Autodesk Inventor part; units mm, degrees
(part 3 of 4)
sketch "Швелер 24" plane through (0, 0, 0) normal (0, 0, 1) x (1, 0, 0)
  line L0 (-3.4674, 143.7463) -> (-3.4674, -55.2537)
  line L1 (80.9326, -75.7537) -> (-9.0674, -75.7537)
  line L2 (-9.0674, -75.7537) -> (-9.0674, 164.2463)
  line L3 (-9.0674, 164.2463) -> (80.9326, 164.2463)
  line L4 (76.9326, 154.2463) -> (7.0326, 154.2463)
  arc A0 (7.0326, 154.2463) -> (-3.4674, 143.7463) centre (7.0326, 143.7463) ccw
  arc A1 (-3.4674, -55.2537) -> (7.0326, -65.7537) centre (7.0326, -55.2537) ccw
  line L5 (7.0326, -65.7537) -> (76.9326, -65.7537)
  line L6 (80.9326, -75.7537) -> (80.9326, -69.7537)
  arc A2 (80.9326, -69.7537) -> (76.9326, -65.7537) centre (76.9326, -69.7537) ccw
  line L7 (80.9326, 164.2463) -> (80.9326, 158.2463)
  arc A3 (76.9326, 154.2463) -> (80.9326, 158.2463) centre (76.9326, 158.2463) ccw
  point P0 (39.2152, 43.3464)
  dimension "d495" = 90
  dimension "d496" = 240
  dimension "d497" = 5.6
  dimension "d498" = 10.5
  dimension "d499" = 4
  dimension "d500" = 10
  measures "d495" distance of L1.start L1.end
  measures "d496" distance of L1.end L2.end
  measures "d497" distance between parallel lines of L2 L0
  measures "d498" radius of A1
  measures "d499" radius of A2
  measures "d500" distance between parallel lines of L1 L5
sketch "Швелер 24а" plane through (0, 0, 0) normal (0, 0, 1) x (1, 0, 0)
  line L0 (-6.1145, 143.0463) -> (-6.1145, -54.5537)
  line L1 (83.2855, -75.7537) -> (-11.7145, -75.7537)
  line L2 (-11.7145, -75.7537) -> (-11.7145, 164.2463)
  line L3 (-11.7145, 164.2463) -> (83.2855, 164.2463)
  line L4 (79.2855, 153.5463) -> (4.3855, 153.5463)
  arc A0 (4.3855, 153.5463) -> (-6.1145, 143.0463) centre (4.3855, 143.0463) ccw
  arc A1 (-6.1145, -54.5537) -> (4.3855, -65.0537) centre (4.3855, -54.5537) ccw
  line L5 (4.3855, -65.0537) -> (79.2855, -65.0537)
  line L6 (83.2855, -75.7537) -> (83.2855, -69.0537)
  arc A2 (83.2855, -69.0537) -> (79.2855, -65.0537) centre (79.2855, -69.0537) ccw
  line L7 (83.2855, 164.2463) -> (83.2855, 157.5463)
  arc A3 (79.2855, 153.5463) -> (83.2855, 157.5463) centre (79.2855, 157.5463) ccw
  point P0 (39.2152, 43.3464)
  dimension "d501" = 95
  dimension "d502" = 240
  dimension "d503" = 5.6
  dimension "d504" = 10.5
  dimension "d505" = 4
  dimension "d506" = 10.7
  measures "d501" distance of L1.start L1.end
  measures "d502" distance of L1.end L2.end
  measures "d503" distance between parallel lines of L2 L0
  measures "d504" radius of A1
  measures "d505" radius of A2
  measures "d506" distance between parallel lines of L1 L5
sketch "Швелер 27" plane through (0, 0, 0) normal (0, 0, 1) x (1, 0, 0)
  line L0 (-5.8322, 157.7463) -> (-5.8322, -69.2537)
  line L1 (83.1678, -90.7537) -> (-11.8322, -90.7537)
  line L2 (-11.8322, -90.7537) -> (-11.8322, 179.2463)
  line L3 (-11.8322, 179.2463) -> (83.1678, 179.2463)
  line L4 (78.6678, 168.7463) -> (5.1678, 168.7463)
  arc A0 (5.1678, 168.7463) -> (-5.8322, 157.7463) centre (5.1678, 157.7463) ccw
  arc A1 (-5.8322, -69.2537) -> (5.1678, -80.2537) centre (5.1678, -69.2537) ccw
  line L5 (5.1678, -80.2537) -> (78.6678, -80.2537)
  line L6 (83.1678, -90.7537) -> (83.1678, -84.7537)
  arc A2 (83.1678, -84.7537) -> (78.6678, -80.2537) centre (78.6678, -84.7537) ccw
  line L7 (83.1678, 179.2463) -> (83.1678, 173.2463)
  arc A3 (78.6678, 168.7463) -> (83.1678, 173.2463) centre (78.6678, 173.2463) ccw
  point P0 (39.2152, 43.3464)
  dimension "d507" = 95
  dimension "d508" = 270
  dimension "d509" = 6
  dimension "d510" = 11
  dimension "d511" = 4.5
  dimension "d512" = 10.5
  measures "d507" distance of L1.start L1.end
  measures "d508" distance of L1.end L2.end
  measures "d509" distance between parallel lines of L2 L0
  measures "d510" radius of A1
  measures "d511" radius of A2
  measures "d512" distance between parallel lines of L1 L5
sketch "Швелер 30" plane through (0, 0, 0) normal (0, 0, 1) x (1, 0, 0)
  line L0 (-8.2439, 171.2463) -> (-8.2439, -82.7537)
  line L1 (85.2561, -105.7537) -> (-14.7439, -105.7537)
  line L2 (-14.7439, -105.7537) -> (-14.7439, 194.2463)
  line L3 (-14.7439, 194.2463) -> (85.2561, 194.2463)
  line L4 (80.2561, 183.2463) -> (3.7561, 183.2463)
  arc A0 (3.7561, 183.2463) -> (-8.2439, 171.2463) centre (3.7561, 171.2463) ccw
  arc A1 (-8.2439, -82.7537) -> (3.7561, -94.7537) centre (3.7561, -82.7537) ccw
  line L5 (3.7561, -94.7537) -> (80.2561, -94.7537)
  line L6 (85.2561, -105.7537) -> (85.2561, -99.7537)
  arc A2 (85.2561, -99.7537) -> (80.2561, -94.7537) centre (80.2561, -99.7537) ccw
  line L7 (85.2561, 194.2463) -> (85.2561, 188.2463)
  arc A3 (80.2561, 183.2463) -> (85.2561, 188.2463) centre (80.2561, 188.2463) ccw
  point P0 (39.2152, 43.3464)
  dimension "d513" = 100
  dimension "d514" = 300
  dimension "d515" = 6.5
  dimension "d516" = 12
  dimension "d517" = 5
  dimension "d518" = 11
  measures "d513" distance of L1.start L1.end
  measures "d514" distance of L1.end L2.end
  measures "d515" distance between parallel lines of L2 L0
  measures "d516" radius of A1
  measures "d517" radius of A2
  measures "d518" distance between parallel lines of L1 L5
sketch "Швелер 33" plane through (0, 0, 0) normal (0, 0, 1) x (1, 0, 0)
  line L0 (-10.7733, 184.5463) -> (-10.7733, -96.0537)
  line L1 (87.2267, -120.7537) -> (-17.7733, -120.7537)
  line L2 (-17.7733, -120.7537) -> (-17.7733, 209.2463)
  line L3 (-17.7733, 209.2463) -> (87.2267, 209.2463)
  line L4 (82.2267, 197.5463) -> (2.2267, 197.5463)
  arc A0 (2.2267, 197.5463) -> (-10.7733, 184.5463) centre (2.2267, 184.5463) ccw
  arc A1 (-10.7733, -96.0537) -> (2.2267, -109.0537) centre (2.2267, -96.0537) ccw
  line L5 (2.2267, -109.0537) -> (82.2267, -109.0537)
  line L6 (87.2267, -120.7537) -> (87.2267, -114.0537)
  arc A2 (87.2267, -114.0537) -> (82.2267, -109.0537) centre (82.2267, -114.0537) ccw
  line L7 (87.2267, 209.2463) -> (87.2267, 202.5463)
  arc A3 (82.2267, 197.5463) -> (87.2267, 202.5463) centre (82.2267, 202.5463) ccw
  point P0 (39.2152, 43.3464)
  dimension "d519" = 105
  dimension "d520" = 330
  dimension "d521" = 7
  dimension "d522" = 13
  dimension "d523" = 5
  dimension "d524" = 11.7
  measures "d519" distance of L1.start L1.end
  measures "d520" distance of L1.end L2.end
  measures "d521" distance between parallel lines of L2 L0
  measures "d522" radius of A1
  measures "d523" radius of A2
  measures "d524" distance between parallel lines of L1 L5
sketch "Швелер 36" plane through (0, 0, 0) normal (0, 0, 1) x (1, 0, 0)
  line L0 (-13.0674, 197.6463) -> (-13.0674, -109.1537)
  line L1 (89.4326, -135.7537) -> (-20.5674, -135.7537)
  line L2 (-20.5674, -135.7537) -> (-20.5674, 224.2463)
  line L3 (-20.5674, 224.2463) -> (89.4326, 224.2463)
  line L4 (83.4326, 211.6463) -> (0.9326, 211.6463)
  arc A0 (0.9326, 211.6463) -> (-13.0674, 197.6463) centre (0.9326, 197.6463) ccw
  arc A1 (-13.0674, -109.1537) -> (0.9326, -123.1537) centre (0.9326, -109.1537) ccw
  line L5 (0.9326, -123.1537) -> (83.4326, -123.1537)
  line L6 (89.4326, -135.7537) -> (89.4326, -129.1537)
  arc A2 (89.4326, -129.1537) -> (83.4326, -123.1537) centre (83.4326, -129.1537) ccw
  line L7 (89.4326, 224.2463) -> (89.4326, 217.6463)
  arc A3 (83.4326, 211.6463) -> (89.4326, 217.6463) centre (83.4326, 217.6463) ccw
  point P0 (39.2152, 43.3464)
  dimension "d525" = 110
  dimension "d526" = 360
  dimension "d527" = 7.5
  dimension "d528" = 14
  dimension "d529" = 6
  dimension "d530" = 12.6
  measures "d525" distance of L1.start L1.end
  measures "d526" distance of L1.end L2.end
  measures "d527" distance between parallel lines of L2 L0
  measures "d528" radius of A1
  measures "d529" radius of A2
  measures "d530" distance between parallel lines of L1 L5
sketch "Швелер 40" plane through (0, 0, 0) normal (0, 0, 1) x (1, 0, 0)
  line L0 (-15.5969, 215.7463) -> (-15.5969, -127.2537)
  line L1 (91.4031, -155.7537) -> (-23.5969, -155.7537)
  line L2 (-23.5969, -155.7537) -> (-23.5969, 244.2463)
  line L3 (-23.5969, 244.2463) -> (91.4031, 244.2463)
  line L4 (85.4031, 230.7463) -> (-0.5969, 230.7463)
  arc A0 (-0.5969, 230.7463) -> (-15.5969, 215.7463) centre (-0.5969, 215.7463) ccw
  arc A1 (-15.5969, -127.2537) -> (-0.5969, -142.2537) centre (-0.5969, -127.2537) ccw
  line L5 (-0.5969, -142.2537) -> (85.4031, -142.2537)
  line L6 (91.4031, -155.7537) -> (91.4031, -148.2537)
  arc A2 (91.4031, -148.2537) -> (85.4031, -142.2537) centre (85.4031, -148.2537) ccw
  line L7 (91.4031, 244.2463) -> (91.4031, 236.7463)
  arc A3 (85.4031, 230.7463) -> (91.4031, 236.7463) centre (85.4031, 236.7463) ccw
  point P0 (39.2152, 43.3464)
  dimension "d531" = 115
  dimension "d532" = 400
  dimension "d533" = 8
  dimension "d534" = 15
  dimension "d535" = 6
  dimension "d536" = 13.5
  measures "d531" distance of L1.start L1.end
  measures "d532" distance of L1.end L2.end
  measures "d533" distance between parallel lines of L2 L0
  measures "d534" radius of A1
  measures "d535" radius of A2
  measures "d536" distance between parallel lines of L1 L5
sketch "Швелер з нахилом 5" plane through (0, 0, 0) normal (0, 0, 1) x (1, 0, 0)
  line L0 (26.3778, 61.5391) -> (26.3778, 38.5788)
  line L1 (53.9778, 25.059) -> (21.9778, 25.059)
  line L2 (21.9778, 25.059) -> (21.9778, 75.059)
  line L3 (21.9778, 75.059) -> (53.9778, 75.059)
  arc A0 (31.9885, 67.5265) -> (26.3778, 61.5391) centre (32.3778, 61.5391) ccw
  arc A1 (26.3778, 38.5788) -> (31.9885, 32.5914) centre (32.3778, 38.5788) ccw
  line L4 (53.9778, 25.059) -> (53.9778, 28.819)
  line L5 (31.9885, 32.5914) -> (51.64, 31.3137)
  arc A2 (53.9778, 28.819) -> (51.64, 31.3137) centre (51.4778, 28.819) ccw
  line L6 (53.9778, 75.059) -> (53.9778, 71.299)
  arc A3 (51.64, 68.8042) -> (53.9778, 71.299) centre (51.4778, 71.299) ccw
  line L7 (51.64, 68.8042) -> (31.9885, 67.5265)
  point P0 (39.2152, 43.3464)
  point P1 (40.1778, 32.059)
  dimension "d537" = 32
  dimension "d538" = 50
  dimension "d540" = 4.4
  dimension "d542" = 6
  dimension "d873" = 3.76
  dimension "d874" = 2.5
  dimension "d875" = 13.8
  dimension "d876" = 7
  measures "d537" distance of L1.start L1.end
  measures "d538" distance of L1.end L2.end
  measures "d540" distance between parallel lines of L2 L0
  measures "d542" radius of A1
  measures "d873" distance of L1.start L4.end
  measures "d874" radius of A2
  measures "d875" horizontal distance of L1.start point (40.178, 32.059)
  measures "d876" distance from line of L1 point (40.178, 32.059)
sketch "Швелер з нахилом 6.5" plane through (0, 0, 0) normal (0, 0, 1) x (1, 0, 0)
  line L0 (70.1087, 96.6719) -> (70.1087, 59.417)
  line L1 (101.7087, 45.5445) -> (65.7087, 45.5445)
  line L2 (65.7087, 45.5445) -> (65.7087, 110.5445)
  line L3 (65.7087, 110.5445) -> (101.7087, 110.5445)
  arc A0 (75.7061, 102.6584) -> (70.1087, 96.6719) centre (76.1087, 96.6719) ccw
  arc A1 (70.1087, 59.417) -> (75.7061, 53.4306) centre (76.1087, 59.417) ccw
  line L4 (101.7087, 45.5445) -> (101.7087, 49.3445)
  line L5 (75.7061, 53.4306) -> (99.3764, 51.8389)
  arc A2 (101.7087, 49.3445) -> (99.3764, 51.8389) centre (99.2087, 49.3445) ccw
  line L6 (101.7087, 110.5445) -> (101.7087, 106.7445)
  arc A3 (99.3764, 104.2501) -> (101.7087, 106.7445) centre (99.2087, 106.7445) ccw
  line L7 (99.3764, 104.2501) -> (75.7061, 102.6584)
  point P0 (39.2152, 43.3464)
  point P1 (85.9087, 52.7445)
  dimension "d877" = 36
  dimension "d878" = 65
  dimension "d879" = 4.4
  dimension "d880" = 6
  dimension "d881" = 3.8
  dimension "d882" = 2.5
  dimension "d883" = 15.8
  dimension "d884" = 7.2
  measures "d877" distance of L4.start L1.end
  measures "d878" distance of L1.end L3.start
  measures "d879" distance between parallel lines of L2 L0
  measures "d880" radius of A1
  measures "d881" distance of L4.start L4.end
  measures "d882" radius of A2
  measures "d883" horizontal distance of L4.start point (85.909, 52.744)
  measures "d884" distance from line of L1 point (85.909, 52.744)
sketch "Швелер з нахилом 8" plane through (0, 0, 0) normal (0, 0, 1) x (1, 0, 0)
  line L0 (22.2355, 76.1423) -> (22.2355, 25.5132)
  line L1 (57.7355, 10.8277) -> (17.7355, 10.8277)
  line L2 (17.7355, 10.8277) -> (17.7355, 90.8277)
  line L3 (17.7355, 90.8277) -> (57.7355, 90.8277)
  arc A0 (28.2915, 82.6271) -> (22.2355, 76.1423) centre (28.7355, 76.1423) ccw
  arc A1 (22.2355, 25.5132) -> (28.2915, 19.0284) centre (28.7355, 25.5132) ccw
  line L4 (57.7355, 10.8277) -> (57.7355, 14.6777)
  line L5 (28.2915, 19.0284) -> (55.4063, 17.1719)
  arc A2 (57.7355, 14.6777) -> (55.4063, 17.1719) centre (55.2355, 14.6777) ccw
  line L6 (57.7355, 90.8277) -> (57.7355, 86.9777)
  arc A3 (55.4063, 84.4836) -> (57.7355, 86.9777) centre (55.2355, 86.9777) ccw
  line L7 (55.4063, 84.4836) -> (28.2915, 82.6271)
  point P0 (39.2152, 43.3464)
  point P1 (39.9855, 18.2277)
  dimension "d885" = 40
  dimension "d886" = 80
  dimension "d887" = 4.5
  dimension "d888" = 6.5
  dimension "d889" = 3.85
  dimension "d890" = 2.5
  dimension "d891" = 17.75
  dimension "d892" = 7.4
  measures "d885" distance of L4.start L1.end
  measures "d886" distance of L1.end L3.start
  measures "d887" distance between parallel lines of L2 L0
  measures "d888" radius of A1
  measures "d889" distance of L4.start L4.end
  measures "d890" radius of A2
  measures "d891" horizontal distance of L4.start point (39.986, 18.228)
  measures "d892" distance from line of L1 point (39.986, 18.228)
sketch "Швелер з нахилом 10" plane through (0, 0, 0) normal (0, 0, 1) x (1, 0, 0)
  line L0 (19.1577, 85.7641) -> (19.1577, 16.9236)
  line L1 (60.6577, 1.3438) -> (14.6577, 1.3438)
  line L2 (14.6577, 1.3438) -> (14.6577, 101.3438)
  line L3 (14.6577, 101.3438) -> (60.6577, 101.3438)
  arc A0 (25.6688, 92.747) -> (19.1577, 85.7641) centre (26.1577, 85.7641) ccw
  arc A1 (19.1577, 16.9236) -> (25.6688, 9.9407) centre (26.1577, 16.9236) ccw
  line L4 (60.6577, 1.3438) -> (60.6577, 4.6938)
  line L5 (25.6688, 9.9407) -> (57.8672, 7.6865)
  arc A2 (60.6577, 4.6938) -> (57.8672, 7.6865) centre (57.6577, 4.6938) ccw
  line L6 (60.6577, 101.3438) -> (60.6577, 97.9938)
  arc A3 (57.8672, 95.0012) -> (60.6577, 97.9938) centre (57.6577, 97.9938) ccw
  line L7 (57.8672, 95.0012) -> (25.6688, 92.747)
  point P0 (39.2152, 43.3464)
  point P1 (39.9077, 8.9438)
  dimension "d893" = 46
  dimension "d894" = 100
  dimension "d895" = 4.5
  dimension "d896" = 7
  dimension "d897" = 3.35
  dimension "d898" = 3
  dimension "d899" = 20.75
  dimension "d900" = 7.6
  measures "d893" distance of L4.start L1.end
  measures "d894" distance of L1.end L3.start
  measures "d895" distance between parallel lines of L2 L0
  measures "d896" radius of A1
  measures "d897" distance of L4.start L4.end
  measures "d898" radius of A2
  measures "d899" horizontal distance of L4.start point (39.908, 8.944)
  measures "d900" distance from line of L1 point (39.908, 8.944)
sketch "Швелер з нахилом 12" plane through (0, 0, 0) normal (0, 0, 1) x (1, 0, 0)
  line L0 (16.5445, 95.4003) -> (16.5445, 8.3241)
  line L1 (63.7445, -8.1378) -> (11.7445, -8.1378)
  line L2 (11.7445, -8.1378) -> (11.7445, 111.8622)
  line L3 (11.7445, 111.8622) -> (63.7445, 111.8622)
  arc A0 (23.5133, 102.8815) -> (16.5445, 95.4003) centre (24.0445, 95.4003) ccw
  arc A1 (16.5445, 8.3241) -> (23.5133, 0.8429) centre (24.0445, 8.3241) ccw
  line L4 (63.7445, -8.1378) -> (63.7445, -4.8078)
  line L5 (23.5133, 0.8429) -> (60.9569, -1.8153)
  arc A2 (63.7445, -4.8078) -> (60.9569, -1.8153) centre (60.7445, -4.8078) ccw
  line L6 (63.7445, 111.8622) -> (63.7445, 108.5322)
  arc A3 (60.9569, 105.5397) -> (63.7445, 108.5322) centre (60.7445, 108.5322) ccw
  line L7 (60.9569, 105.5397) -> (23.5133, 102.8815)
  point P0 (39.2152, 43.3464)
  point P1 (40.1445, -0.3378)
  dimension "d901" = 52
  dimension "d902" = 120
  dimension "d903" = 4.8
  dimension "d904" = 7.5
  dimension "d905" = 3.33
  dimension "d906" = 3
  dimension "d907" = 23.6
  dimension "d908" = 7.8
  measures "d901" distance of L4.start L1.end
  measures "d902" distance of L1.end L3.start
  measures "d903" distance between parallel lines of L2 L0
  measures "d904" radius of A1
  measures "d905" distance of L4.start L4.end
  measures "d906" radius of A2
  measures "d907" horizontal distance of L4.start point (40.144, -0.338)
  measures "d908" distance from line of L1 point (40.144, -0.338)
sketch "Швелер з нахилом 14" plane through (0, 0, 0) normal (0, 0, 1) x (1, 0, 0)
  line L0 (119.2067, 148.6254) -> (119.2067, 43.5326)
  line L1 (172.3067, 26.079) -> (114.3067, 26.079)
  line L2 (114.3067, 26.079) -> (114.3067, 166.079)
  line L3 (114.3067, 166.079) -> (172.3067, 166.079)
  arc A0 (126.6333, 156.6048) -> (119.2067, 148.6254) centre (127.2067, 148.6254) ccw
  arc A1 (119.2067, 43.5326) -> (126.6333, 35.5532) centre (127.2067, 43.5326) ccw
  line L4 (172.3067, 26.079) -> (172.3067, 29.479)
  line L5 (126.6333, 35.5532) -> (169.5217, 32.4713)
  arc A2 (172.3067, 29.479) -> (169.5217, 32.4713) centre (169.3067, 29.479) ccw
  line L6 (172.3067, 166.079) -> (172.3067, 162.679)
  arc A3 (169.5217, 159.6867) -> (172.3067, 162.679) centre (169.3067, 162.679) ccw
  line L7 (169.5217, 159.6867) -> (126.6333, 156.6048)
  point P0 (39.2152, 43.3464)
  point P1 (145.7567, 34.179)
  dimension "d909" = 58
  dimension "d910" = 140
  dimension "d911" = 4.9
  dimension "d912" = 8
  dimension "d913" = 3.4
  dimension "d914" = 3
  dimension "d915" = 26.55
  dimension "d916" = 8.1
  measures "d909" distance of L4.start L1.end
  measures "d910" distance of L1.end L3.start
  measures "d911" distance between parallel lines of L2 L0
  measures "d912" radius of A1
  measures "d913" distance of L4.start L4.end
  measures "d914" radius of A2
  measures "d915" horizontal distance of L4.start point (145.757, 34.179)
  measures "d916" distance from line of L1 point (145.757, 34.179)
sketch "Швелер з нахилом 14а" plane through (0, 0, 0) normal (0, 0, 1) x (1, 0, 0)
  line L0 (10.9429, 103.7671) -> (10.9429, 0.9116)
  line L1 (68.0429, -17.6606) -> (6.0429, -17.6606)
  line L2 (6.0429, -17.6606) -> (6.0429, 122.3394)
  line L3 (6.0429, 122.3394) -> (68.0429, 122.3394)
  arc A0 (18.2294, 111.7352) -> (10.9429, 103.7671) centre (18.9429, 103.7671) ccw
  arc A1 (10.9429, 0.9116) -> (18.2294, -7.0565) centre (18.9429, 0.9116) ccw
  line L4 (68.0429, -17.6606) -> (68.0429, -14.2606)
  line L5 (18.2294, -7.0565) -> (65.3105, -11.2726)
  arc A2 (68.0429, -14.2606) -> (65.3105, -11.2726) centre (65.0429, -14.2606) ccw
  line L6 (68.0429, 122.3394) -> (68.0429, 118.9394)
  arc A3 (65.3105, 115.9513) -> (68.0429, 118.9394) centre (65.0429, 118.9394) ccw
  line L7 (65.3105, 115.9513) -> (18.2294, 111.7352)
  point P0 (39.2152, 43.3464)
  point P1 (39.4929, -8.9606)
  dimension "d917" = 62
  dimension "d918" = 140
  dimension "d919" = 4.9
  dimension "d920" = 8
  dimension "d921" = 3.4
  dimension "d922" = 3
  dimension "d923" = 28.55
  dimension "d924" = 8.7
  measures "d917" distance of L4.start L1.end
  measures "d918" distance of L1.end L3.start
  measures "d919" distance between parallel lines of L2 L0
  measures "d920" radius of A1
  measures "d921" distance of L4.start L4.end
  measures "d922" radius of A2
  measures "d923" horizontal distance of L4.start point (39.493, -8.961)
  measures "d924" distance from line of L1 point (39.493, -8.961)
sketch "Швелер з нахилом 16" plane through (0, 0, 0) normal (0, 0, 1) x (1, 0, 0)
  line L0 (10.0678, 114.4401) -> (10.0678, -8.6771)
  line L1 (69.0678, -27.1185) -> (5.0678, -27.1185)
  line L2 (5.0678, -27.1185) -> (5.0678, 132.8815)
  line L3 (5.0678, 132.8815) -> (69.0678, 132.8815)
  arc A0 (17.9545, 122.918) -> (10.0678, 114.4401) centre (18.5678, 114.4401) ccw
  arc A1 (10.0678, -8.6771) -> (17.9545, -17.155) centre (18.5678, -8.6771) ccw
  line L4 (69.0678, -27.1185) -> (69.0678, -24.1085)
  line L5 (17.9545, -17.155) -> (65.8203, -20.6176)
  arc A2 (69.0678, -24.1085) -> (65.8203, -20.6176) centre (65.5678, -24.1085) ccw
  line L6 (69.0678, 132.8815) -> (69.0678, 129.8715)
  arc A3 (65.8203, 126.3806) -> (69.0678, 129.8715) centre (65.5678, 129.8715) ccw
  line L7 (65.8203, 126.3806) -> (17.9545, 122.918)
  point P0 (39.2152, 43.3464)
  point P1 (39.5678, -18.7185)
  dimension "d925" = 64
  dimension "d926" = 160
  dimension "d927" = 5
  dimension "d928" = 8.5
  dimension "d929" = 3.01
  dimension "d930" = 3.5
  dimension "d931" = 29.5
  dimension "d932" = 8.4
  measures "d925" distance of L4.start L1.end
  measures "d926" distance of L1.end L3.start
  measures "d927" distance between parallel lines of L2 L0
  measures "d928" radius of A1
  measures "d929" distance of L4.start L4.end
  measures "d930" radius of A2
  measures "d931" horizontal distance of L4.start point (39.568, -18.719)
  measures "d932" distance from line of L1 point (39.568, -18.719)
sketch "Швелер з нахилом 16а" plane through (0, 0, 0) normal (0, 0, 1) x (1, 0, 0)
  line L0 (70.9587, -27.1501) -> (70.9587, -23.7001)
  arc A0 (70.9587, -23.7001) -> (67.7131, -20.2094) centre (67.4587, -23.7001) ccw
  line L1 (15.8408, -16.4288) -> (67.7131, -20.2094)
  arc A1 (7.9587, -7.9512) -> (15.8408, -16.4288) centre (16.4587, -7.9512) ccw
  line L2 (70.9587, -27.1501) -> (2.9587, -27.1501)
  arc A2 (67.7131, 125.9092) -> (70.9587, 129.3999) centre (67.4587, 129.3999) ccw
  line L3 (70.9587, 132.8499) -> (70.9587, 129.3999)
  line L4 (7.9587, 113.6511) -> (7.9587, -7.9512)
  line L5 (67.7131, 125.9092) -> (15.8408, 122.1286)
  line L6 (2.9587, 132.8499) -> (70.9587, 132.8499)
  arc A3 (15.8408, 122.1286) -> (7.9587, 113.6511) centre (16.4587, 113.6511) ccw
  line L7 (2.9587, -27.1501) -> (2.9587, 132.8499)
  point P0 (39.2152, 43.3464)
  point P1 (39.4587, -18.1501)
  dimension "d933" = 68
  dimension "d934" = 160
  dimension "d935" = 5
  dimension "d936" = 8.5
  dimension "d937" = 3.45
  dimension "d938" = 3.5
  dimension "d939" = 31.5
  dimension "d940" = 9
  measures "d933" distance of L0.start L7.start
  measures "d934" distance of L7.start L7.end
  measures "d935" distance between parallel lines of L7 L4
  measures "d936" radius of A1
  measures "d937" distance of L0.start L0.end
  measures "d938" radius of A0
  measures "d939" horizontal distance of L0.start point (39.459, -18.15)
  measures "d940" distance from line of L2 point (39.459, -18.15)
sketch "Швелер з нахилом 18" plane through (0, 0, 0) normal (0, 0, 1) x (1, 0, 0)
  line L0 (71.9498, -36.6077) -> (71.9498, -33.5277)
  arc A0 (71.9498, -33.5277) -> (68.7043, -30.037) centre (68.4498, -33.5277) ccw
  line L1 (14.9318, -26.1165) -> (68.7043, -30.037)
  arc A1 (7.0498, -17.639) -> (14.9318, -26.1165) centre (15.5498, -17.639) ccw
  line L2 (71.9498, -36.6077) -> (1.9498, -36.6077)
  arc A2 (68.7043, 136.8216) -> (71.9498, 140.3123) centre (68.4498, 140.3123) ccw
  line L3 (71.9498, 143.3923) -> (71.9498, 140.3123)
  line L4 (7.0498, 124.4236) -> (7.0498, -17.639)
  line L5 (68.7043, 136.8216) -> (14.9318, 132.9011)
  line L6 (1.9498, 143.3923) -> (71.9498, 143.3923)
  arc A3 (14.9318, 132.9011) -> (7.0498, 124.4236) centre (15.5498, 124.4236) ccw
  line L7 (1.9498, -36.6077) -> (1.9498, 143.3923)
  point P0 (39.2152, 43.3464)
  point P1 (39.4998, -27.9077)
  dimension "d941" = 70
  dimension "d942" = 180
  dimension "d943" = 5.1
  dimension "d944" = 8.5
  dimension "d945" = 3.08
  dimension "d946" = 3.5
  dimension "d947" = 32.45
  dimension "d948" = 8.7
  measures "d941" distance of L0.start L7.start
  measures "d942" distance of L7.start L7.end
  measures "d943" distance between parallel lines of L7 L4
  measures "d944" radius of A1
  measures "d945" distance of L0.start L0.end
  measures "d946" radius of A0
  measures "d947" horizontal distance of L0.start point (39.5, -27.908)
  measures "d948" distance from line of L2 point (39.5, -27.908)
sketch "Швелер з нахилом 18а" plane through (0, 0, 0) normal (0, 0, 1) x (1, 0, 0)
  line L0 (4.8392, 123.1694) -> (4.8392, -16.448)
  line L1 (-0.2608, -36.6393) -> (-0.2608, 143.3607)
  line L2 (70.4953, 136.3501) -> (13.1807, 132.1453)
  arc A0 (70.4953, 136.3501) -> (73.7392, 139.8407) centre (70.2392, 139.8407) ccw
  line L3 (73.7392, 143.3607) -> (73.7392, 139.8407)
  line L4 (-0.2608, 143.3607) -> (73.7392, 143.3607)
  arc A1 (13.1807, 132.1453) -> (4.8392, 123.1694) centre (13.8392, 123.1694) ccw
  line L5 (13.1807, -25.4239) -> (70.4953, -29.6287)
  arc A2 (73.7392, -33.1193) -> (70.4953, -29.6287) centre (70.2392, -33.1193) ccw
  line L6 (73.7392, -36.6393) -> (73.7392, -33.1193)
  line L7 (73.7392, -36.6393) -> (-0.2608, -36.6393)
  arc A3 (4.8392, -16.448) -> (13.1807, -25.4239) centre (13.8392, -16.448) ccw
  point P0 (39.2152, 43.3464)
  point P1 (39.2892, -27.3393)
  dimension "d949" = 74
  dimension "d950" = 180
  dimension "d951" = 5.1
  dimension "d952" = 9
  dimension "d953" = 3.52
  dimension "d954" = 3.5
  dimension "d955" = 34.45
  dimension "d956" = 9.3
  measures "d949" distance of L7.start L1.start
  measures "d950" distance of L1.start L1.end
  measures "d951" distance between parallel lines of L1 L0
  measures "d952" radius of A3
  measures "d953" distance of L7.start L6.end
  measures "d954" radius of A2
  measures "d955" horizontal distance of L7.start point (39.289, -27.339)
  measures "d956" distance from line of L7 point (39.289, -27.339)
sketch "Швелер з нахилом 20" plane through (0, 0, 0) normal (0, 0, 1) x (1, 0, 0)
  line L0 (3.9277, 133.4727) -> (3.9277, -25.6665)
  line L1 (-1.2723, -46.0969) -> (-1.2723, 153.9031)
  line L2 (71.021, 147.2339) -> (12.7309, 142.9471)
  arc A0 (71.021, 147.2339) -> (74.7277, 151.2231) centre (70.7277, 151.2231) ccw
  line L3 (74.7277, 153.9031) -> (74.7277, 151.2231)
  line L4 (-1.2723, 153.9031) -> (74.7277, 153.9031)
  arc A1 (12.7309, 142.9471) -> (3.9277, 133.4727) centre (13.4277, 133.4727) ccw
  line L5 (12.7309, -35.1409) -> (71.021, -39.4277)
  arc A2 (74.7277, -43.4169) -> (71.021, -39.4277) centre (70.7277, -43.4169) ccw
  line L6 (74.7277, -46.0969) -> (74.7277, -43.4169)
  line L7 (74.7277, -46.0969) -> (-1.2723, -46.0969)
  arc A3 (3.9277, -25.6665) -> (12.7309, -35.1409) centre (13.4277, -25.6665) ccw
  point P0 (39.2152, 43.3464)
  point P1 (39.3277, -37.0969)
  dimension "d957" = 76
  dimension "d958" = 200
  dimension "d959" = 5.2
  dimension "d960" = 9.5
  dimension "d961" = 2.68
  dimension "d962" = 4
  dimension "d963" = 35.4
  dimension "d964" = 9
  measures "d957" distance of L7.start L1.start
  measures "d958" distance of L1.start L1.end
  measures "d959" distance between parallel lines of L1 L0
  measures "d960" radius of A3
  measures "d961" distance of L7.start L6.end
  measures "d962" radius of A2
  measures "d963" horizontal distance of L7.start point (39.328, -37.097)
  measures "d964" distance from line of L7 point (39.328, -37.097)
sketch "Швелер з нахилом 20а" plane through (0, 0, 0) normal (0, 0, 1) x (1, 0, 0)
  line L0 (1.8371, 132.1188) -> (1.8371, -24.3861)
  line L1 (-3.3629, -46.1337) -> (-3.3629, 153.8663)
  line L2 (72.9954, 147.2024) -> (10.4862, 141.5806)
  arc A0 (72.9954, 147.2024) -> (76.6371, 151.1863) centre (72.6371, 151.1863) ccw
  line L3 (76.6371, 153.8663) -> (76.6371, 151.1863)
  line L4 (-3.3629, 153.8663) -> (76.6371, 153.8663)
  arc A1 (10.4862, 141.5806) -> (1.8371, 132.1188) centre (11.3371, 132.1188) ccw
  line L5 (10.4862, -33.8479) -> (72.9954, -39.4697)
  arc A2 (76.6371, -43.4537) -> (72.9954, -39.4697) centre (72.6371, -43.4537) ccw
  line L6 (76.6371, -46.1337) -> (76.6371, -43.4537)
  line L7 (76.6371, -46.1337) -> (-3.3629, -46.1337)
  arc A3 (1.8371, -24.3861) -> (10.4862, -33.8479) centre (11.3371, -24.3861) ccw
  point P0 (39.2152, 43.3464)
  point P1 (39.2371, -36.4337)
  dimension "d965" = 80
  dimension "d966" = 200
  dimension "d967" = 5.2
  dimension "d968" = 9.5
  dimension "d969" = 2.68
  dimension "d970" = 4
  dimension "d971" = 37.4
  dimension "d972" = 9.7
  measures "d965" distance of L7.start L1.start
  measures "d966" distance of L1.start L1.end
  measures "d967" distance between parallel lines of L1 L0
  measures "d968" radius of A3
  measures "d969" distance of L7.start L6.end
  measures "d970" radius of A2
  measures "d971" horizontal distance of L7.start point (39.237, -36.434)
  measures "d972" distance from line of L7 point (39.237, -36.434)
sketch "Швелер з нахилом 22" plane through (0, 0, 0) normal (0, 0, 1) x (1, 0, 0)
  line L0 (0.8857, 142.7895) -> (0.8857, -33.9827)
  line L1 (-4.5143, -55.5966) -> (-4.5143, 164.4034)
  line L2 (73.7799, 157.4542) -> (10.1504, 152.7625)
  arc A0 (73.7799, 157.4542) -> (77.4857, 161.4434) centre (73.4857, 161.4434) ccw
  line L3 (77.4857, 164.4034) -> (77.4857, 161.4434)
  line L4 (-4.5143, 164.4034) -> (77.4857, 164.4034)
  arc A1 (10.1504, 152.7625) -> (0.8857, 142.7895) centre (10.8857, 142.7895) ccw
  line L5 (10.1504, -43.9557) -> (73.7799, -48.6474)
  arc A2 (77.4857, -52.6366) -> (73.7799, -48.6474) centre (73.4857, -52.6366) ccw
  line L6 (77.4857, -55.5966) -> (77.4857, -52.6366)
  line L7 (77.4857, -55.5966) -> (-4.5143, -55.5966)
  arc A3 (0.8857, -33.9827) -> (10.1504, -43.9557) centre (10.8857, -33.9827) ccw
  point P0 (39.2152, 43.3464)
  point P1 (39.1857, -46.0966)
  dimension "d973" = 82
  dimension "d974" = 220
  dimension "d975" = 5.4
  dimension "d976" = 10
  dimension "d977" = 2.96
  dimension "d978" = 4
  dimension "d979" = 38.3
  dimension "d980" = 9.5
  measures "d973" distance of L7.start L1.start
  measures "d974" distance of L1.start L1.end
  measures "d975" distance between parallel lines of L1 L0
  measures "d976" radius of A3
  measures "d977" distance of L7.start L6.end
  measures "d978" radius of A2
  measures "d979" horizontal distance of L7.start point (39.186, -46.097)
  measures "d980" distance from line of L7 point (39.186, -46.097)
sketch "Швелер з нахилом 22а" plane through (0, 0, 0) normal (0, 0, 1) x (1, 0, 0)
  line L0 (-7.1435, -55.6335) -> (-7.1435, 164.3665)
  line L1 (-1.7435, 141.4293) -> (-1.7435, -32.6962)
  arc A0 (-1.7435, -32.6962) -> (7.3835, -42.6581) centre (8.2565, -32.6962) ccw
  line L2 (7.3835, -42.6581) -> (76.2056, -48.6887)
  line L3 (79.8565, -55.6335) -> (-7.1435, -55.6335)
  arc A1 (79.8565, -52.6735) -> (76.2056, -48.6887) centre (75.8565, -52.6735) ccw
  line L4 (79.8565, -55.6335) -> (79.8565, -52.6735)
  arc A2 (7.3835, 151.3911) -> (-1.7435, 141.4293) centre (8.2565, 141.4293) ccw
  line L5 (76.2056, 157.4218) -> (7.3835, 151.3911)
  line L6 (-7.1435, 164.3665) -> (79.8565, 164.3665)
  arc A3 (76.2056, 157.4218) -> (79.8565, 161.4065) centre (75.8565, 161.4065) ccw
  line L7 (79.8565, 164.3665) -> (79.8565, 161.4065)
  point P0 (39.2152, 43.3464)
  point P1 (39.0565, -45.4335)
  dimension "d981" = 87
  dimension "d982" = 220
  dimension "d983" = 5.4
  dimension "d984" = 10
  dimension "d985" = 2.96
  dimension "d986" = 4
  dimension "d987" = 40.8
  dimension "d988" = 10.2
  measures "d981" distance of L4.start L3.end
  measures "d982" distance of L3.end L0.end
  measures "d983" distance between parallel lines of L0 L1
  measures "d984" radius of A0
  measures "d985" distance of L4.start L4.end
  measures "d986" radius of A1
  measures "d987" horizontal distance of L4.start point (39.056, -45.433)
  measures "d988" distance from line of L3 point (39.056, -45.433)
sketch "Швелер з нахилом 24" plane through (0, 0, 0) normal (0, 0, 1) x (1, 0, 0)
  line L0 (61.9989, -53.6873) -> (61.9989, 186.3127)
  line L1 (67.5989, 163.4362) -> (67.5989, -30.8109)
  arc A0 (67.5989, -30.8109) -> (77.3234, -41.2823) centre (78.0989, -30.8109) ccw
  line L2 (77.3234, -41.2823) -> (148.2943, -46.5383)
  line L3 (151.9989, -53.6873) -> (61.9989, -53.6873)
  arc A1 (151.9989, -50.5273) -> (148.2943, -46.5383) centre (147.9989, -50.5273) ccw
  line L4 (151.9989, -53.6873) -> (151.9989, -50.5273)
  arc A2 (77.3234, 173.9076) -> (67.5989, 163.4362) centre (78.0989, 163.4362) ccw
  line L5 (148.2943, 179.1636) -> (77.3234, 173.9076)
  line L6 (61.9989, 186.3127) -> (151.9989, 186.3127)
  arc A3 (148.2943, 179.1636) -> (151.9989, 183.1527) centre (147.9989, 183.1527) ccw
  line L7 (151.9989, 186.3127) -> (151.9989, 183.1527)
  point P0 (39.2152, 43.3464)
  point P1 (109.7989, -43.6873)
  dimension "d989" = 90
  dimension "d990" = 240
  dimension "d991" = 5.6
  dimension "d992" = 10.5
  dimension "d993" = 3.16
  dimension "d994" = 4
  dimension "d995" = 42.2
  dimension "d996" = 10
  measures "d989" distance of L4.start L3.end
  measures "d990" distance of L3.end L0.end
  measures "d991" distance between parallel lines of L0 L1
  measures "d992" radius of A0
  measures "d993" distance of L4.start L4.end
  measures "d994" radius of A1
  measures "d995" horizontal distance of L4.start point (109.799, -43.687)
  measures "d996" distance from line of L3 point (109.799, -43.687)
sketch "Швелер з нахилом 24а" plane through (0, 0, 0) normal (0, 0, 1) x (1, 0, 0)
  arc A0 (154.3697, -50.5642) -> (150.7149, -46.5791) centre (150.3697, -50.5642) ccw
  line L0 (154.3697, -53.7242) -> (154.3697, -50.5642)
  arc A1 (64.9697, -29.5228) -> (74.5637, -39.9837) centre (75.4697, -29.5228) ccw
  line L1 (74.5637, -39.9837) -> (150.7149, -46.5791)
  line L2 (154.3697, -53.7242) -> (59.3697, -53.7242)
  line L3 (64.9697, 162.0744) -> (64.9697, -29.5228)
  line L4 (59.3697, -53.7242) -> (59.3697, 186.2758)
  arc A2 (74.5637, 172.5353) -> (64.9697, 162.0744) centre (75.4697, 162.0744) ccw
  line L5 (150.7149, 179.1307) -> (74.5637, 172.5353)
  line L6 (59.3697, 186.2758) -> (154.3697, 186.2758)
  arc A3 (150.7149, 179.1307) -> (154.3697, 183.1158) centre (150.3697, 183.1158) ccw
  line L7 (154.3697, 186.2758) -> (154.3697, 183.1158)
  point P0 (39.2152, 43.3464)
  point P1 (109.6697, -43.0242)
  dimension "d997" = 95
  dimension "d998" = 240
  dimension "d999" = 5.6
  dimension "d1000" = 10.5
  dimension "d1001" = 3.16
  dimension "d1002" = 4
  dimension "d1003" = 44.7
  dimension "d1004" = 10.7
  measures "d997" distance of L2.start L4.start
  measures "d998" distance of L4.start L4.end
  measures "d999" distance between parallel lines of L4 L3
  measures "d1000" radius of A1
  measures "d1001" distance of L2.start L0.end
  measures "d1002" radius of A0
  measures "d1003" horizontal distance of L2.start point (109.67, -43.024)
  measures "d1004" distance from line of L2 point (109.67, -43.024)
sketch "Швелер з нахилом 27" plane through (0, 0, 0) normal (0, 0, 1) x (1, 0, 0)
  arc A0 (154.3526, -64.8938) -> (150.1844, -60.406) centre (149.8526, -64.8938) ccw
  line L0 (154.3526, -67.9238) -> (154.3526, -64.8938)
  arc A1 (65.3526, -43.9166) -> (75.5414, -54.8867) centre (76.3526, -43.9166) ccw
  line L1 (75.5414, -54.8867) -> (150.1844, -60.406)
  line L2 (154.3526, -67.9238) -> (59.3526, -67.9238)
  line L3 (65.3526, 178.0691) -> (65.3526, -43.9166)
  line L4 (59.3526, -67.9238) -> (59.3526, 202.0762)
  arc A2 (75.5414, 189.0392) -> (65.3526, 178.0691) centre (76.3526, 178.0691) ccw
  line L5 (150.1844, 194.5585) -> (75.5414, 189.0392)
  line L6 (59.3526, 202.0762) -> (154.3526, 202.0762)
  arc A3 (150.1844, 194.5585) -> (154.3526, 199.0462) centre (149.8526, 199.0462) ccw
  line L7 (154.3526, 202.0762) -> (154.3526, 199.0462)
  point P0 (39.2152, 43.3464)
  point P1 (109.8526, -57.4238)
  dimension "d1005" = 95
  dimension "d1006" = 270
  dimension "d1007" = 6
  dimension "d1008" = 11
  dimension "d1009" = 3.03
  dimension "d1010" = 4.5
  dimension "d1011" = 44.5
  dimension "d1012" = 10.5
  measures "d1005" distance of L2.start L4.start
  measures "d1006" distance of L4.start L4.end
  measures "d1007" distance between parallel lines of L4 L3
  measures "d1008" radius of A1
  measures "d1009" distance of L2.start L0.end
  measures "d1010" radius of A0
  measures "d1011" horizontal distance of L2.start point (109.853, -57.424)
  measures "d1012" distance from line of L2 point (109.853, -57.424)
sketch "Швелер з нахилом 30" plane through (0, 0, 0) normal (0, 0, 1) x (1, 0, 0)
  arc A0 (156.5754, -79.2602) -> (151.944, -74.2738) centre (151.5754, -79.2602) ccw
  line L0 (156.5754, -82.1602) -> (156.5754, -79.2602)
  arc A1 (63.0754, -56.5585) -> (74.1907, -68.5259) centre (75.0754, -56.5585) ccw
  line L1 (74.1907, -68.5259) -> (151.944, -74.2738)
  line L2 (156.5754, -82.1602) -> (56.5754, -82.1602)
  line L3 (63.0754, 192.2382) -> (63.0754, -56.5585)
  line L4 (56.5754, -82.1602) -> (56.5754, 217.8398)
  arc A2 (74.1907, 204.2056) -> (63.0754, 192.2382) centre (75.0754, 192.2382) ccw
  line L5 (151.944, 209.9534) -> (74.1907, 204.2056)
  line L6 (56.5754, 217.8398) -> (156.5754, 217.8398)
  arc A3 (151.944, 209.9534) -> (156.5754, 214.9398) centre (151.5754, 214.9398) ccw
  line L7 (156.5754, 217.8398) -> (156.5754, 214.9398)
  point P0 (39.2152, 43.3464)
  point P1 (109.8254, -71.1602)
  dimension "d1013" = 100
  dimension "d1014" = 300
  dimension "d1015" = 6.5
  dimension "d1016" = 12
  dimension "d1017" = 2.9
  dimension "d1018" = 5
  dimension "d1019" = 46.75
  dimension "d1020" = 11
  measures "d1013" distance of L2.start L4.start
  measures "d1014" distance of L4.start L4.end
  measures "d1015" distance between parallel lines of L4 L3
  measures "d1016" radius of A1
  measures "d1017" distance of L2.start L0.end
  measures "d1018" radius of A0
  measures "d1019" horizontal distance of L2.start point (109.825, -71.16)
  measures "d1020" distance from line of L2 point (109.825, -71.16)
sketch "Швелер з нахилом 33" plane through (0, 0, 0) normal (0, 0, 1) x (1, 0, 0)
  arc A0 (158.695, -92.9671) -> (154.0629, -87.9807) centre (153.695, -92.9671) ccw
  line L0 (158.695, -96.4071) -> (158.695, -92.9671)
  arc A1 (60.695, -69.0156) -> (72.7385, -81.9804) centre (73.695, -69.0156) ccw
  line L1 (72.7385, -81.9804) -> (154.0629, -87.9807)
  line L2 (158.695, -96.4071) -> (53.695, -96.4071)
  line L3 (60.695, 206.2014) -> (60.695, -69.0156)
  line L4 (53.695, -96.4071) -> (53.695, 233.5929)
  arc A2 (72.7385, 219.1662) -> (60.695, 206.2014) centre (73.695, 206.2014) ccw
  line L5 (154.0629, 225.1665) -> (72.7385, 219.1662)
  line L6 (53.695, 233.5929) -> (158.695, 233.5929)
  arc A3 (154.0629, 225.1665) -> (158.695, 230.1529) centre (153.695, 230.1529) ccw
  line L7 (158.695, 233.5929) -> (158.695, 230.1529)
  point P0 (39.2152, 43.3464)
  point P1 (109.695, -84.7071)
  dimension "d1021" = 105
  dimension "d1022" = 330
  dimension "d1023" = 7
  dimension "d1024" = 13
  dimension "d1025" = 3.44
  dimension "d1026" = 5
  dimension "d1027" = 49
  dimension "d1028" = 11.7
  measures "d1021" distance of L2.start L4.start
  measures "d1022" distance of L4.start L4.end
  measures "d1023" distance between parallel lines of L4 L3
  measures "d1024" radius of A1
  measures "d1025" distance of L2.start L0.end
  measures "d1026" radius of A0
  measures "d1027" horizontal distance of L2.start point (109.695, -84.707)
  measures "d1028" distance from line of L2 point (109.695, -84.707)
sketch "Швелер з нахилом 36" plane through (0, 0, 0) normal (0, 0, 1) x (1, 0, 0)
  arc A0 (161.0143, -107.4046) -> (155.4538, -101.4207) centre (155.0143, -107.4046) ccw
  line L0 (161.0143, -110.6646) -> (161.0143, -107.4046)
  arc A1 (58.5143, -81.2907) -> (71.4887, -95.2531) centre (72.5143, -81.2907) ccw
  line L1 (71.4887, -95.2531) -> (155.4538, -101.4207)
  line L2 (161.0143, -110.6646) -> (51.0143, -110.6646)
  line L3 (58.5143, 219.9615) -> (58.5143, -81.2907)
  line L4 (51.0143, -110.6646) -> (51.0143, 249.3354)
  arc A2 (71.4887, 233.9239) -> (58.5143, 219.9615) centre (72.5143, 219.9615) ccw
  line L5 (155.4538, 240.0915) -> (71.4887, 233.9239)
  line L6 (51.0143, 249.3354) -> (161.0143, 249.3354)
  arc A3 (155.4538, 240.0915) -> (161.0143, 246.0754) centre (155.0143, 246.0754) ccw
  line L7 (161.0143, 249.3354) -> (161.0143, 246.0754)
  point P0 (39.2152, 43.3464)
  point P1 (109.7643, -98.0646)
  dimension "d1029" = 110
  dimension "d1030" = 360
  dimension "d1031" = 7.5
  dimension "d1032" = 14
  dimension "d1033" = 3.26
  dimension "d1034" = 6
  dimension "d1035" = 51.25
  dimension "d1036" = 12.6
  measures "d1029" distance of L2.start L4.start
  measures "d1030" distance of L4.start L4.end
  measures "d1031" distance between parallel lines of L4 L3
  measures "d1032" radius of A1
  measures "d1033" distance of L2.start L0.end
  measures "d1034" radius of A0
  measures "d1035" horizontal distance of L2.start point (109.764, -98.065)
  measures "d1036" distance from line of L2 point (109.764, -98.065)
sketch "Швелер з нахилом 40" plane through (0, 0, 0) normal (0, 0, 1) x (1, 0, 0)
  arc A0 (163.0032, -125.6593) -> (157.4421, -119.6754) centre (157.0032, -125.6593) ccw
  line L0 (163.0032, -129.6593) -> (163.0032, -125.6593)
  arc A1 (56.0032, -98.2952) -> (69.9059, -113.2551) centre (71.0032, -98.2952) ccw
  line L1 (69.9059, -113.2551) -> (157.4421, -119.6754)
  line L2 (163.0032, -129.6593) -> (48.0032, -129.6593)
  line L3 (56.0032, 238.9766) -> (56.0032, -98.2952)
  line L4 (48.0032, -129.6593) -> (48.0032, 270.3407)
  arc A2 (69.9059, 253.9364) -> (56.0032, 238.9766) centre (71.0032, 238.9766) ccw
  line L5 (157.4421, 260.3568) -> (69.9059, 253.9364)
  line L6 (48.0032, 270.3407) -> (163.0032, 270.3407)
  arc A3 (157.4421, 260.3568) -> (163.0032, 266.3407) centre (157.0032, 266.3407) ccw
  line L7 (163.0032, 270.3407) -> (163.0032, 266.3407)
  point P0 (39.2152, 43.3464)
  point P1 (109.5032, -116.1593)
  dimension "d1037" = 115
  dimension "d1038" = 400
  dimension "d1039" = 8
  dimension "d1040" = 15
  dimension "d1041" = 4
  dimension "d1042" = 6
  dimension "d1043" = 53.5
  dimension "d1044" = 13.5
  measures "d1037" distance of L2.start L4.start
  measures "d1038" distance of L4.start L4.end
  measures "d1039" distance between parallel lines of L4 L3
  measures "d1040" radius of A1
  measures "d1041" distance of L2.start L0.end
  measures "d1042" radius of A0
  measures "d1043" horizontal distance of L2.start point (109.503, -116.159)
  measures "d1044" distance from line of L2 point (109.503, -116.159)
sketch "Двотавр 10" plane through (0, 0, 0) normal (0, 0, 1) x (1, 0, 0)
  arc A0 (264.1428, 249.161) -> (257.836, 256.1266) centre (257.1428, 249.161) ccw
  arc A1 (274.9496, 256.1266) -> (268.6428, 249.161) centre (275.6428, 249.161) ccw
  arc A2 (257.836, 171.7842) -> (264.1428, 178.7498) centre (257.1428, 178.7498) ccw
  arc A3 (268.6428, 178.7498) -> (274.9496, 171.7842) centre (275.6428, 178.7498) ccw
  line L0 (238.8928, 163.9554) -> (293.8928, 163.9554)
  line L1 (268.6428, 178.7498) -> (268.6428, 249.161)
  line L2 (293.8928, 263.9554) -> (238.8928, 263.9554)
  line L3 (264.1428, 249.161) -> (264.1428, 178.7498)
  line L4 (274.9496, 256.1266) -> (291.6404, 257.7877)
  arc A4 (291.6404, 257.7877) -> (293.8928, 260.2754) centre (291.3928, 260.2754) ccw
  line L5 (293.8928, 260.2754) -> (293.8928, 263.9554)
  line L6 (257.836, 256.1266) -> (241.1452, 257.7877)
  arc A5 (238.8928, 260.2754) -> (241.1452, 257.7877) centre (241.3928, 260.2754) ccw
  line L7 (238.8928, 260.2754) -> (238.8928, 263.9554)
  line L8 (257.836, 171.7842) -> (241.1452, 170.1231)
  arc A6 (241.1452, 170.1231) -> (238.8928, 167.6354) centre (241.3928, 167.6354) ccw
  line L9 (238.8928, 167.6354) -> (238.8928, 163.9554)
  line L10 (293.8928, 163.9554) -> (293.8928, 167.6354)
  arc A7 (293.8928, 167.6354) -> (291.6404, 170.1231) centre (291.3928, 167.6354) ccw
  line L11 (291.6404, 170.1231) -> (274.9496, 171.7842)
  point P0 (262.5027, 203.4372)
  point P1 (266.3928, 263.9554)
  point P2 (266.3928, 163.9554)
  point P3 (281.2678, 171.1554)
  dimension "d712" = 100
  dimension "d713" = 55
  dimension "d714" = 4.5
  dimension "d718" = 7
  dimension "d1045" = 2.5
  dimension "d1046" = 3.68
  dimension "d1047" = 12.625
  dimension "d1048" = 7.2
  measures "d712" distance between parallel lines of L0 L2
  measures "d713" distance of L0.start L0.end
  measures "d714" distance between parallel lines of L3 L1
  measures "d718" radius of A3
  measures "d1045" radius of A7
  measures "d1046" distance of L0.end L10.end
  measures "d1047" horizontal distance of L0.end point (281.268, 171.155)
  measures "d1048" distance from line of L0 point (281.268, 171.155)
sketch "Двотавр 12" plane through (0, 0, 0) normal (0, 0, 1) x (1, 0, 0)
  arc A0 (63.7598, 210.6116) -> (57.003, 218.0746) centre (56.2598, 210.6116) ccw
  arc A1 (75.3165, 218.0746) -> (68.5598, 210.6116) centre (76.0598, 210.6116) ccw
  arc A2 (57.003, 114.2767) -> (63.7598, 121.7398) centre (56.2598, 121.7398) ccw
  arc A3 (68.5598, 121.7398) -> (75.3165, 114.2767) centre (76.0598, 121.7398) ccw
  line L0 (34.1598, 106.1757) -> (98.1598, 106.1757)
  line L1 (68.5598, 121.7398) -> (68.5598, 210.6116)
  line L2 (98.1598, 226.1757) -> (34.1598, 226.1757)
  line L3 (63.7598, 210.6116) -> (63.7598, 121.7398)
  line L4 (75.3165, 218.0746) -> (95.4571, 220.0804)
  arc A4 (95.4571, 220.0804) -> (98.1598, 223.0657) centre (95.1598, 223.0657) ccw
  line L5 (98.1598, 223.0657) -> (98.1598, 226.1757)
  line L6 (57.003, 218.0746) -> (36.8625, 220.0804)
  arc A5 (34.1598, 223.0657) -> (36.8625, 220.0804) centre (37.1598, 223.0657) ccw
  line L7 (34.1598, 223.0657) -> (34.1598, 226.1757)
  line L8 (57.003, 114.2767) -> (36.8625, 112.2709)
  arc A6 (36.8625, 112.2709) -> (34.1598, 109.2857) centre (37.1598, 109.2857) ccw
  line L9 (34.1598, 109.2857) -> (34.1598, 106.1757)
  line L10 (98.1598, 106.1757) -> (98.1598, 109.2857)
  arc A7 (98.1598, 109.2857) -> (95.4571, 112.2709) centre (95.1598, 109.2857) ccw
  line L11 (95.4571, 112.2709) -> (75.3165, 114.2767)
  point P0 (262.5027, 203.4372)
  point P1 (66.1598, 226.1757)
  point P2 (66.1598, 106.1757)
  point P3 (83.3598, 113.4757)
  dimension "d1049" = 120
  dimension "d1050" = 64
  dimension "d1051" = 4.8
  dimension "d1052" = 7.5
  dimension "d1053" = 3
  dimension "d1054" = 3.11
  dimension "d1055" = 14.8
  dimension "d1056" = 7.3
  measures "d1049" distance between parallel lines of L0 L2
  measures "d1050" distance of L0.start L0.end
  measures "d1051" distance between parallel lines of L3 L1
  measures "d1052" radius of A3
  measures "d1053" radius of A7
  measures "d1054" distance of L0.end L10.end
  measures "d1055" horizontal distance of L0.end point (83.36, 113.476)
  measures "d1056" distance from line of L0 point (83.36, 113.476)
sketch "Двотавр 14" plane through (0, 0, 0) normal (0, 0, 1) x (1, 0, 0)
  arc A0 (264.2379, 267.5463) -> (257.0298, 275.507) centre (256.2379, 267.5463) ccw
  arc A1 (276.3459, 275.507) -> (269.1379, 267.5463) centre (277.1379, 267.5463) ccw
  arc A2 (257.0298, 152.4602) -> (264.2379, 160.4209) centre (256.2379, 160.4209) ccw
  arc A3 (269.1379, 160.4209) -> (276.3459, 152.4602) centre (277.1379, 160.4209) ccw
  line L0 (230.1879, 143.9836) -> (303.1879, 143.9836)
  line L1 (269.1379, 160.4209) -> (269.1379, 267.5463)
  line L2 (303.1879, 283.9836) -> (230.1879, 283.9836)
  line L3 (264.2379, 267.5463) -> (264.2379, 160.4209)
  line L4 (276.3459, 275.507) -> (300.4848, 277.9083)
  arc A4 (300.4848, 277.9083) -> (303.1879, 280.8936) centre (300.1879, 280.8936) ccw
  line L5 (303.1879, 280.8936) -> (303.1879, 283.9836)
  line L6 (257.0298, 275.507) -> (232.8909, 277.9083)
  arc A5 (230.1879, 280.8936) -> (232.8909, 277.9083) centre (233.1879, 280.8936) ccw
  line L7 (230.1879, 280.8936) -> (230.1879, 283.9836)
  line L8 (257.0298, 152.4602) -> (232.8909, 150.0588)
  arc A6 (232.8909, 150.0588) -> (230.1879, 147.0736) centre (233.1879, 147.0736) ccw
  line L9 (230.1879, 147.0736) -> (230.1879, 143.9836)
  line L10 (303.1879, 143.9836) -> (303.1879, 147.0736)
  arc A7 (303.1879, 147.0736) -> (300.4848, 150.0588) centre (300.1879, 147.0736) ccw
  line L11 (300.4848, 150.0588) -> (276.3459, 152.4602)
  point P0 (262.5027, 203.4372)
  point P1 (266.6879, 283.9836)
  point P2 (266.6879, 143.9836)
  point P3 (286.1629, 151.4836)
  dimension "d1057" = 140
  dimension "d1058" = 73
  dimension "d1059" = 4.9
  dimension "d1060" = 8
  dimension "d1061" = 3
  dimension "d1062" = 3.09
  dimension "d1063" = 17.025
  dimension "d1064" = 7.5
  measures "d1057" distance between parallel lines of L0 L2
  measures "d1058" distance of L0.start L0.end
  measures "d1059" distance between parallel lines of L3 L1
  measures "d1060" radius of A3
  measures "d1061" radius of A7
  measures "d1062" distance of L0.end L10.end
  measures "d1063" horizontal distance of L0.end point (286.163, 151.484)
  measures "d1064" distance from line of L0 point (286.163, 151.484)